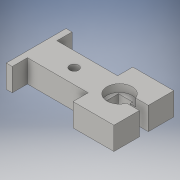
# Autodesk Inventor part: Maglev_holder
Saved by Autodesk Inventor 2016 (Build 200138000, 138)
## iProperties
Created: 2018-01-06
Part Number: Maglev_holder
Material: Generic
Document SubType Name: Modeling
Designer: Jorian Bruslind
Density: 1 g/cm^3
Appearance: Default
Author: Jorian Bruslind
Autodesk Inventor part; units mm, degrees
ref_plane "YZ Plane" through (0, 0, 0) normal (1, 0, 0) x (0, 1, 0)
ref_plane "XZ Plane" through (0, 0, 0) normal (0, 1, 0) x (-1, 0, 0)
ref_plane "XY Plane" through (0, 0, 0) normal (0, 0, 1) x (1, 0, 0)
sketch "Sketch1" plane through (0, 0, 0) normal (0, 1, 0) x (-1, 0, 0)
  line L0 (0, 0) -> (-90, 0)
  line L1 (-90, 0) -> (-90, -50)
  line L2 (-90, -50) -> (0, -50)
  line L3 (0, -50) -> (0, 0)
  line L4 (0, 0) -> (-5, 0)
  line L5 (0, -50) -> (-5, -50)
  line L6 (-5, -50) -> (-5, -37.3)
  line L7 (-5, 0) -> (-5, -12.7)
  line L8 (-5, -12.7) -> (-55.8, -12.7)
  line L9 (-55.8, -12.7) -> (-55.8, 0)
  line L10 (-55.8, 0) -> (-5, 0)
  line L11 (-5, 0) -> (-5, -12.7)
  line L12 (-5, -37.3) -> (-55.8, -37.3)
  line L13 (-55.8, -37.3) -> (-55.8, -50)
  line L14 (-55.8, -50) -> (-5, -50)
  line L15 (-5, -50) -> (-5, -37.3)
  dimension "d0" = 90
  dimension "d1" = 50
  dimension "d4" = 5
  dimension "d5" = 5
  dimension "d6" = 12.7
  dimension "d7" = 12.7
  dimension "d8" = 50.8
  dimension "d9" = 12.7
  dimension "d10" = 50.8
  dimension "d11" = 12.7
  constraints: 32 end point, 6 parallel, 4 perpendicular, 3 horizontal, 2 point on line, 1 vertical
  measures "d0" distance of L2.end L1.end
  measures "d1" distance of L1.end L0.end
  measures "d4" distance of L0.start L4.end
  measures "d5" distance of L2.end L5.end
  measures "d6" distance of L5.end L6.end
  measures "d7" distance of L4.end L7.end
  measures "d8" distance of L9.end L10.end
  measures "d9" distance of L8.end L9.end
  measures "d10" distance of L14.end L13.end
  measures "d11" distance of L13.end L12.end
extrude "Extrusion2" add sketch "Sketch1" along normal blind 19.05 contours L3 L2 L6 L12 L13 L1 L0 L9 L8 L7
sketch "Sketch3" plane through (0, 19.05, 0) normal (0, 1, 0) x (1, 0, 0)
  line L0 (90, 0) -> (90, 50) projected
  line L1 (90, 25) -> (74.76, 25)
  line L2 (90, 25) -> (90, 28.75)
  line L3 (90, 25) -> (90, 21.2408)
  line L4 (90, 21.2408) -> (74.76, 21.2408)
  line L5 (74.76, 21.2408) -> (74.76, 28.7408)
  line L6 (74.76, 28.7408) -> (90, 28.7408)
  line L7 (90, 28.7408) -> (90, 21.2408)
  point P0 (0, 0)
  dimension "d18" = 15.24
  dimension "d19" = 3.75
  dimension "d20" = 3.7592
  dimension "d21" = 15.24
  dimension "d22" = 7.5
  constraints: 14 end point, 2 horizontal, 2 parallel, 2 point on line, 1 midpoint, 1 perpendicular
  measures "d18" distance of L1.start L1.end
  measures "d19" distance of L1.start L2.end
  measures "d20" distance of L1.start L3.end
  measures "d21" distance of L5.end L6.end
  measures "d22" distance of L4.end L5.end
extrude "Extrusion4" cut sketch "Sketch3" against normal blind 19.05
sketch "Sketch4" plane through (0, 19.05, 0) normal (0, 1, 0) x (1, 0, 0)
  line L0 (74.76, 28.7408) -> (74.76, 21.2408) projected
  line L1 (74.76, 24.9908) -> (74.76, 30.9852)
  line L2 (74.76, 30.9852) -> (62.76, 30.9852)
  line L3 (62.76, 30.9852) -> (62.76, 18.9964)
  line L4 (62.76, 18.9964) -> (74.76, 18.9964)
  line L5 (74.76, 18.9964) -> (74.76, 30.9852)
  point P0 (0, 0)
  dimension "d25" = 5.9944
  dimension "d26" = 12
  dimension "d27" = 11.9888
  constraints: 10 end point, 2 parallel, 1 horizontal, 1 midpoint, 1 perpendicular, 1 point on line
  measures "d25" distance of L1.start L1.end
  measures "d26" distance of L4.end L3.end
  measures "d27" distance of L3.end L2.end
extrude "Extrusion5" cut sketch "Sketch4" against normal blind 19.05
sketch "Sketch5" plane through (0, 19.05, 0) normal (0, 1, 0) x (1, 0, 0)
  circle A0 centre (69.68, 24.9908) radius 10.5
  point P0 (0, 0)
  dimension "d30" = 21
  constraints: 1 centre point
  measures "d30" diameter of A0
extrude "Extrusion6" cut sketch "Sketch5" against normal blind 6.35
sketch "Sketch6" plane through (0, 19.05, 0) normal (0, 1, 0) x (1, 0, 0)
  line L0 (0, 50) -> (0, 0) projected
  line L1 (0, 25) -> (31.75, 25)
  circle A0 centre (31.75, 25) radius 3.75
  dimension "d33" = 31.75
  dimension "d34" = 7.5
  constraints: 2 end point, 1 centre point, 1 coincident, 1 horizontal, 1 midpoint
  measures "d33" distance of L1.start L1.end
  measures "d34" diameter of A0
extrude "Extrusion7" cut sketch "Sketch6" against normal blind 19.05
body "Solid2"
